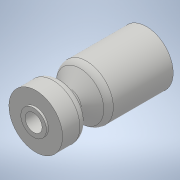
# Autodesk Inventor part: Подпорный
Saved by Autodesk Inventor 2020 (Build 240168000, 168)
## iProperties
Created: 2021-05-10
Part Number: Подпорный
Material: Типовые
Document SubType Name: Modeling
Designer: I_Love_U_Bogdan
Density: 1 g/cm^3
Appearance: По умолчанию
Author: I_Love_U_Bogdan
Autodesk Inventor part; units mm, degrees
ref_plane "YZ Plane" through (0, 0, 0) normal (1, 0, 0) x (0, 1, 0)
ref_plane "XZ Plane" through (0, 0, 0) normal (0, 1, 0) x (-1, 0, 0)
ref_plane "XY Plane" through (0, 0, 0) normal (0, 0, 1) x (1, 0, 0)
sketch "Эскиз1" plane through (0, 0, 0) normal (0, 0, 1) x (1, 0, 0)
  circle A0 centre (59.7064, -71.2479) radius 6.3
  line L0 (59.7064, -64.9479) -> (59.7064, -77.5479)
  point P0 (0, 0)
  dimension "d0" = 12.6
  constraints: 2 end point, 2 point on circle, 1 centre point, 1 vertical
  measures "d0" diameter of A0
extrude "Выдавливание1" add sketch "Эскиз1" along normal blind 26 contours L0 A0 picked at (58.2279, -73.1684)
sketch "Эскиз2" plane through (59.7064, -71.2479, 26) normal (0, 0, 1) x (0, -1, 0)
  circle A0 centre (0, 0) radius 3
  point P0 (-71.2479, -59.7064)
  dimension "d3" = 6
  constraints: 1 centre point
  measures "d3" diameter of A0
extrude "Выдавливание2" add sketch "Эскиз2" along normal blind 0.5
sketch "Эскиз3" plane through (59.7064, -71.2479, 26.5) normal (0, 0, 1) x (1, 0, 0)
  circle A0 centre (0, 0) radius 2
  point P0 (-59.7064, 71.2479)
  dimension "d6" = 4
  constraints: 1 centre point
  measures "d6" diameter of A0
extrude "Выдавливание3" cut sketch "Эскиз3" against normal through all
sketch "Эскиз4" plane through (59.7064, -77.5479, 26) normal (1, 0, 0) x (0, 0, -1)
  line L0 (11, 0) -> (11, 4.3)
  line L1 (26, 4.3) -> (0, 4.3) projected
  line L2 (26, 0) -> (26, 4.3) projected
  line L3 (5, 4.3) -> (5, 0)
  line L4 (26, 0) -> (0, 0) projected
  line L5 (26, 12.6) -> (26, 0) projected
  line L6 (26, 6.3) -> (-3.2365, 6.3)
  line L7 (8, 0) -> (8, 4.3)
  line L8 (11, 0) -> (8, 3.5753)
  line L9 (11, 0) -> (11.1053, 0) construction
  line L10 (8, 3.5753) -> (5, 0)
  point P0 (26, 77.5479)
  dimension "d9" = 15
  dimension "d10" = 6
  dimension "d11" = 3
  dimension "d12" = 130
  dimension "d15" = 3.5753
  constraints: 14 end point, 7 point on line, 2 horizontal, 2 perpendicular, 2 vertical, 1 midpoint
  measures "d9" distance between parallel lines of L2 L0
  measures "d10" distance between parallel lines of L0 L3
  measures "d11" distance between parallel lines of L3 L7
  measures "d12" angle of L9 L8
  measures "d15" distance of L7.start L8.end
revolve "Вращение1" cut sketch "Эскиз4" angle 360 about axis through (59.7064, -71.2479, 0) along (0, 0, 1) contours L4 L7 L8 | L4 L10 L7
fillet "Сопряжение1" radius 2 2 edges at (53.4064, -71.2479, 15) (53.4064, -71.2479, 21)
mirror "Зеркальное отражение1" about plane through (59.7064, -77.5479, 0) normal (1, 0, 0)
equation "\"d11\" = 0.5 * d10"
